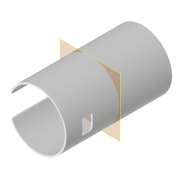
# Autodesk Inventor part: Planktoscope_connectortube
Saved by Autodesk Inventor 2022 (Build 260153000, 153)
## iProperties
Created: 2022-12-09
Part Number: Planktoscope_connectortube
Material: Generisch
Document SubType Name: Modeling
Designer: diederichbenedict
Density: 1 g/cm^3
Appearance: Vorgabe
Author: diederichbenedict
Autodesk Inventor part; units mm, degrees
ref_plane "YZ Plane" through (0, 0, 0) normal (1, 0, 0) x (0, 1, 0)
ref_plane "XZ Plane" through (0, 0, 0) normal (0, 1, 0) x (-1, 0, 0)
ref_plane "XY Plane" through (0, 0, 0) normal (0, 0, 1) x (1, 0, 0)
ref_plane "Arbeitsebene1" through (0, 0, 0) normal (0, 0, 1) x (1, 0, 0)
sketch "Skizze1" plane through (0, 0, 0) normal (0, 0, 1) x (1, 0, 0)
  circle A0 centre (0, 0.5522) radius 27.7
  circle A1 centre (0, 0.5522) radius 26.2
  point P0 (0, 0)
  dimension "d11" = 52.4
  dimension "d12" = 55.4
  constraints: 2 centre point, 1 coincident
  measures "d11" diameter of A1
  measures "d12" diameter of A0
extrude "Extrusion1" add sketch "Skizze1" along normal mid plane 100
sketch "Skizze3" plane through (0, 0, 0) normal (1, 0, 0) x (0, 1, 0)
  line L0 (-27.1478, -50) -> (-27.1478, 50) projected
  line L1 (28.2522, -50) -> (28.2522, 50) projected
  line L2 (9.2777, 59.671) -> (-10.7223, 59.671)
  line L3 (-10.7223, 59.671) -> (-10.7223, -5)
  line L4 (-10.7223, -5) -> (9.2777, -5)
  line L5 (9.2777, -5) -> (9.2777, 59.671)
  line L6 (9.2777, 59.671) -> (-10.7223, -5) construction
  line L7 (-10.7223, 59.671) -> (9.2777, -5) construction
  line L8 (0.5522, 50) -> (0.5522, 50) projected
  point P0 (0, 0)
  point P1 (-0.7223, 27.3355)
  dimension "d13" = 20
  dimension "d14" = 55
  constraints: 12 end point, 2 midpoint, 2 parallel, 1 horizontal, 1 perpendicular
  measures "d13" distance of L4.end L3.end
  measures "d14" distance between parallel lines of L8 L4
extrude "Extrusion3" cut sketch "Skizze3" against normal blind 75
fillet "Rundung1" radius 2 4 edges at (-25.4971, 9.2777, 50) (-25.4971, 9.2777, -5) (-24.4759, -10.7223, 50) (-24.4759, -10.7223, -5)
sketch "Skizze4" plane through (0, 0, 0) normal (1, 0, 0) x (0, 1, 0)
  line L0 (-10.7223, 48) -> (-10.7223, -3) projected
  line L1 (-8.7223, -5) -> (7.2777, -5) projected
  line L2 (9.2777, -3) -> (9.2777, 48) projected
  line L3 (-12.7223, 50) -> (11.2777, 50) projected
  line L4 (-27.1478, -50) -> (28.2522, -50) projected
  line L5 (5.5, 35) -> (-5.5, 35)
  line L6 (-7.5, 33) -> (-7.5, 27)
  line L7 (-5.5, 25) -> (5.5, 25)
  line L8 (7.5, 27) -> (7.5, 33)
  line L9 (7.5, 35) -> (-7.5, 25) construction
  line L10 (-7.5, 35) -> (7.5, 25) construction
  line L11 (-25.6478, 50) -> (26.7522, 50) projected
  line L12 (-2.9499, 34.5) -> (4.0501, 34.5) projected
  arc A0 (7.5, 33) -> (5.5, 35) centre (5.5, 33) ccw
  arc A1 (-5.5, 35) -> (-7.5, 33) centre (-5.5, 33) ccw
  arc A2 (-7.5, 27) -> (-5.5, 25) centre (-5.5, 27) ccw
  arc A3 (5.5, 25) -> (7.5, 27) centre (5.5, 27) ccw
  point P0 (0, 0)
  point P1 (0, 30)
  dimension "d18" = 15
  dimension "d19" = 10
  dimension "d20" = 15
  dimension "d21" = 2
  constraints: 12 end point, 8 point on circle, 8 point on line, 8 tangent, 4 centre point, 3 equal radius, 2 midpoint, 2 parallel, 1 horizontal, 1 perpendicular, 4 other
  measures "d18" distance of L9.start L10.start
  measures "d19" distance of L9.end L10.start
  measures "d20" distance between parallel lines of L5 L3
  measures "d21" radius of A0
extrude "Extrusion4" cut sketch "Skizze4" along normal through all
